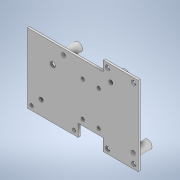
# Autodesk Inventor part: 10_Holder_Step_Down
Saved by Autodesk Inventor 2021 (Build 250183000, 183)
## iProperties
Created: 2021-07-29
Part Number: 10_Holder_Step_Down
Material: Generisch
Document SubType Name: Modeling
Designer: User
Density: 1 g/cm^3
Appearance: Vorgabe
Author: User
Autodesk Inventor part; units mm, degrees
ref_plane "YZ Plane" through (0, 0, 0) normal (1, 0, 0) x (0, 1, 0)
ref_plane "Arbeitsebene1" through (0, 0, 10) normal (0, 0, 1) x (1, 0, 0)
sketch "Skizze1" plane through (0, 0, 10) normal (0, 0, 1) x (1, 0, 0)
  circle A0 centre (19, -33.7337) radius 2 projected
  circle A1 centre (37, -73.7337) radius 2 projected
  circle A2 centre (-37, -73.7337) radius 2 projected
  circle A3 centre (-19, -33.7337) radius 2 projected
  circle A4 centre (37.3592, -81.4668) radius 1.25 projected
  circle A5 centre (16.3592, -81.4668) radius 1.25 projected
  circle A6 centre (16.3592, -24.9668) radius 1.25 projected
  circle A7 centre (37.3592, -24.9668) radius 1.25 projected
  circle A8 centre (9.1592, -42.7989) radius 0.8 projected
  circle A9 centre (-3.6408, -42.7989) radius 0.8 projected
  circle A10 centre (-3.6408, -70.7989) radius 0.8 projected
  circle A11 centre (9.1592, -70.7989) radius 0.8 projected
  circle A12 centre (-44.8022, -81.878) radius 1 projected
  circle A13 centre (-10.6794, -81.878) radius 1 projected
  circle A14 centre (-27.7408, -44.8166) radius 1.5 projected
  line L0 (40.9592, -85.0668) -> (40.9592, -21.3668)
  line L1 (40.9592, -21.3668) -> (12.7592, -21.3668)
  line L2 (12.7592, -21.3668) -> (12.7592, -29.3166)
  line L3 (12.7592, -29.3166) -> (-48.2408, -29.3166)
  line L4 (-48.2408, -29.3166) -> (-48.2408, -85.3166)
  line L5 (40.9592, -85.0668) -> (12.7592, -85.0668)
  line L6 (12.7592, -85.0668) -> (12.7592, -75.3989)
  line L7 (12.7592, -75.3989) -> (-7.2408, -75.3989)
  line L8 (-7.2408, -75.3989) -> (-7.2408, -85.3166)
  line L9 (-7.2408, -85.3166) -> (-48.2408, -85.3166)
  line L10 (39.9592, -84.0668) -> (39.9592, -22.3668) projected
  line L11 (39.9592, -22.3668) -> (13.7592, -22.3668) projected
  line L12 (13.7592, -84.0668) -> (39.9592, -84.0668) projected
  line L13 (13.7592, -22.3668) -> (13.7592, -84.0668) projected
  line L14 (-7.2408, -74.3989) -> (12.7592, -74.3989) projected
  line L15 (-47.2408, -84.3166) -> (-8.2408, -84.3166) projected
  line L16 (-47.2408, -37.3166) -> (-47.2408, -84.3166) projected
  line L17 (-31.0408, -31.3166) -> (-46.2408, -31.3166) projected
  line L18 (-8.2408, -84.3166) -> (-8.2408, -37.3166) projected
  circle A15 centre (-44.8022, -81.878) radius 1
  circle A16 centre (-27.7408, -44.8166) radius 1.7
  circle A17 centre (-3.6408, -42.7989) radius 1
  circle A18 centre (9.1592, -42.7989) radius 1
  circle A19 centre (-10.6794, -81.878) radius 1
  circle A20 centre (-3.6408, -70.7989) radius 1
  circle A21 centre (9.1592, -70.7989) radius 1
  circle A22 centre (16.3592, -81.4668) radius 1.45
  circle A23 centre (37.3592, -81.4668) radius 1.45
  circle A24 centre (37.3592, -24.9668) radius 1.45
  circle A25 centre (16.3592, -24.9668) radius 1.45
  circle A26 centre (19, -33.7337) radius 1.5753
  circle A27 centre (-19, -33.7337) radius 1.5753
  circle A28 centre (37, -73.7337) radius 1.5753
  circle A29 centre (-37, -73.7337) radius 1.5753
  point P0 (0, 0)
  dimension "d0" = 1
  dimension "d1" = 1
  dimension "d2" = 1
  dimension "d3" = 1
  dimension "d4" = 1
  dimension "d5" = 1
  dimension "d6" = 1
  dimension "d7" = 2
  dimension "d8" = 1
  dimension "d9" = 1
  dimension "d18" = 2
  dimension "d19" = 0.2
  dimension "d20" = 0.2
  dimension "d21" = 0.2
  dimension "d22" = 2
  dimension "d23" = 2
  dimension "d24" = 2
  dimension "d25" = 2
  dimension "d26" = 2
  dimension "d27" = 0.2
  dimension "d28" = 0.2
  dimension "d29" = 3.1505
  constraints: 20 end point, 15 centre point, 15 coincident, 8 perpendicular, 3 equal radius, 1 horizontal, 1 vertical
  measures "d0" distance between parallel lines of L0 L10
  measures "d1" distance between parallel lines of L5 L12
  measures "d2" distance between parallel lines of L13 L6
  measures "d3" distance between parallel lines of L14 L7
  measures "d4" distance between parallel lines of L8 L18
  measures "d5" distance between parallel lines of L9 L15
  measures "d6" distance between parallel lines of L16 L4
  measures "d7" distance between parallel lines of L17 L3
  measures "d8" distance between parallel lines of L13 L2
  measures "d9" distance between parallel lines of L11 L1
  measures "d18" diameter of A15
  measures "d19" radial gap between concentric circles of A14 A16
  measures "d20" radial gap between concentric circles of A6 A25
  measures "d21" radial gap between concentric circles of A7 A24
  measures "d22" diameter of A19
  measures "d23" diameter of A17
  measures "d24" diameter of A20
  measures "d25" diameter of A21
  measures "d26" diameter of A18
  measures "d27" radial gap between concentric circles of A5 A22
  measures "d28" radial gap between concentric circles of A4 A23
  measures "d29" diameter of A26
extrude "Extrusion1" add sketch "Skizze1" along normal blind 1.6 contours A0 | A1 | A2 | A3 | L5 L6 L7 L8 L9 L4 L3 L2 L1 L0 | L12 L13 L11 L10
sketch "Skizze2" plane through (0, 0, 10) normal (0, 0, -1) x (-1, 0, 0)
  circle A0 centre (-19, -33.7337) radius 3.4952
  circle A1 centre (19, -33.7337) radius 3.4952
  line L0 (-40.9592, -85.0668) -> (-40.9592, -21.3668) projected
  circle A2 centre (-19, -33.7337) radius 1.5752 projected
  circle A3 centre (19, -33.7337) radius 1.5752 projected
  circle A4 centre (-37, -73.7337) radius 3.4952
  circle A5 centre (-37, -73.7337) radius 1.5752 projected
  circle A6 centre (37, -73.7337) radius 1.5752 projected
  circle A7 centre (37, -73.7337) radius 3.4952
  circle A8 centre (-19, -33.7337) radius 1.5752 projected
  circle A9 centre (19, -33.7337) radius 1.5752 projected
  point P0 (0, 0)
  dimension "d30" = 1.92
  dimension "d31" = 1.92
  dimension "d32" = 1.92
  dimension "d33" = 1.92
  constraints: 8 coincident, 4 centre point
  measures "d30" radial gap between concentric circles of A0 A2
  measures "d31" radial gap between concentric circles of A3 A1
  measures "d32" radial gap between concentric circles of A4 A5
  measures "d33" radial gap between concentric circles of A7 A6
extrude "Extrusion2" add sketch "Skizze2" along normal blind 10
ref_plane "Arbeitsebene2" through (0, 0, -10) normal (0.8937807, 0.4485042, 0) x (0, 0, 1)
chamfer "Fase1" distance 0.5 angle 45 4 edges at (38.5753, -73.7337, 0) (20.5753, -33.7337, 0) (-17.4248, -33.7337, 0) (-35.4248, -73.7337, 0)
sketch "Skizze6" plane through (37, -73.7337, 0) normal (0, 0, -1) x (-1, 0, 0)
  circle A0 centre (0, 0) radius 3.4952 projected
  circle A1 centre (18, 40) radius 3.4952 projected
  circle A2 centre (56, 40) radius 3.4952 projected
  circle A3 centre (74, 0) radius 3.4952 projected
  circle A4 centre (56, 40) radius 1.5752 projected
  circle A5 centre (18, 40) radius 1.5752 projected
  point P0 (37, 73.7337)
  constraints: 4 coincident
sketch "Skizze5" plane through (0, 0, -10) normal (0.8937807, 0.4485042, 0) x (0, 0, 1)
  line L0 (9.55, 84.0717) -> (9.7375, 84.3964)
  line L1 (9.7375, 84.3964) -> (9.8125, 84.3964)
  line L2 (9.8125, 84.3964) -> (10, 84.0717)
  line L3 (10, 84.0717) -> (10.075, 84.0717)
  line L4 (10.15, 84.0717) -> (10.15, 84.4614) construction
  line L5 (10.15, 84.4614) -> (9.4, 84.4614) construction
  line L6 (9.4, 84.4614) -> (9.4, 84.0717) construction
  line L7 (9.4, 84.0717) -> (9.475, 84.0717) construction
  line L8 (9.475, 84.0717) -> (9.55, 84.0717)
  line L9 (10.075, 84.0717) -> (10.15, 84.0717) construction
  line L10 (9.55, 84.0717) -> (10, 84.0717) construction
  line L11 (9.7375, 84.3964) -> (9.775, 84.4614) construction
  line L12 (9.8125, 84.3964) -> (9.775, 84.4614) construction
  line L13 (9.4, 82.4964) -> (10.15, 82.4964) construction
  line L14 (9.4, 84.0717) -> (9.475, 83.9418) construction
  line L15 (9.475, 83.9418) -> (9.55, 84.0717) construction
  line L16 (10, 84.0717) -> (10.075, 83.9418) construction
  line L17 (10.075, 83.9418) -> (10.15, 84.0717) construction
  line L18 (9.775, 84.0717) -> (9.775, 84.4614) construction
  line L19 (9.475, 83.9418) -> (10.075, 83.9418) construction
  line L20 (9.4, 82.4964) -> (9.4, 84.0717) construction
  line L21 (10.15, 82.4964) -> (10.15, 84.0717) construction
  line L22 (9.55, 84.0717) -> (10, 84.0717)
  line L23 (25.04, 82.4964) -> (0.96, 82.4964) projected
  line L24 (10, 80.9212) -> (10, 84.0717) projected
  dimension "d34" = 60
  dimension "d35" = 3.8
  dimension "d36" = 0.6
  dimension "d37" = 3.1505
  dimension "d38" = 0.3247
  dimension "d39" = 0.0649
  constraints: 46 end point, 11 collinear, 5 parallel, 3 midpoint, 3 perpendicular, 3 point on line, 2 coincident, 1 horizontal, 9 other
  measures "d34" angle of L0 L2
  measures "d35" diameter of L0.end L13
  measures "d36" distance of L7.end L3.end
  measures "d37" diameter of L7.end L13
  measures "d38" distance between parallel lines of L1 L10
  measures "d39" distance from line of L18.end L1
coil "Spirale1" sketch "Skizze5" operation cut axis through (37, -73.7337, 10) along (0, 0, 1) pitch 0.6 turns 16.666667 hand right
pattern_sketch "Skizzenbasierte Anordnung1" of "Spirale1" from (37, -73.7337, 0) copies at (-19, -33.7337, 0) at (19, -33.7337, 0) at (-37, -73.7337, 0)
chamfer "Fase2" distance 0.4 angle 45 22 edges at (35.9092, -81.4668, 10) (35.9092, -81.4668, 11.6) (35.9092, -24.9668, 10) (35.9092, -24.9668, 11.6) (14.9092, -81.4668, 10) (14.9092, -81.4668, 11.6) (8.1592, -70.7989, 10) (8.1592, -70.7989, 11.6) (-4.6408, -70.7989, 10) (-4.6408, -70.7989, 11.6) (-11.6794, -81.878, 10) (-11.6794, -81.878, 11.6) (-4.6408, -42.7989, 10) (-4.6408, -42.7989, 11.6) (8.1592, -42.7989, 10) (8.1592, -42.7989, 11.6) (-45.8022, -81.878, 10) (-45.8022, -81.878, 11.6) (-29.4408, -44.8166, 10) (-29.4408, -44.8166, 11.6) (14.9092, -24.9668, 11.6) (14.9092, -24.9668, 10)
sketch "Skizze7" plane through (0, 0, 11.6) normal (0, 0, 1) x (1, 0, 0)
  circle A0 centre (37.3592, -24.9668) radius 1.45 projected
  circle A1 centre (16.3592, -24.9668) radius 1.45 projected
  circle A2 centre (9.1592, -42.7989) radius 1 projected
  circle A3 centre (-3.6408, -42.7989) radius 1 projected
  circle A4 centre (-27.7408, -44.8166) radius 1.7 projected
  circle A5 centre (-3.6408, -70.7989) radius 1 projected
  circle A6 centre (9.1592, -70.7989) radius 1 projected
  circle A7 centre (16.3592, -81.4668) radius 1.45 projected
  circle A8 centre (37.3592, -81.4668) radius 1.45 projected
  circle A9 centre (-10.6794, -81.878) radius 1 projected
  circle A10 centre (-44.8022, -81.878) radius 1 projected
  circle A11 centre (37.3592, -24.9668) radius 2.45
  circle A12 centre (37.3592, -81.4668) radius 2.45
  circle A13 centre (16.3592, -81.4668) radius 1.45 projected
  circle A14 centre (16.3592, -81.4668) radius 2.45
  circle A15 centre (9.1592, -70.7989) radius 1 projected
  circle A16 centre (9.1592, -70.7989) radius 2
  circle A17 centre (9.1592, -42.7989) radius 2
  circle A18 centre (-3.6408, -42.7989) radius 2
  circle A19 centre (-3.6408, -70.7989) radius 2
  circle A20 centre (-44.8022, -81.878) radius 2
  circle A21 centre (-10.6794, -81.878) radius 1 projected
  circle A22 centre (-10.6794, -81.878) radius 2
  circle A23 centre (-27.7408, -44.8166) radius 2.7
  circle A24 centre (16.3592, -24.9668) radius 1.45 projected
  circle A25 centre (16.3592, -24.9668) radius 2.45
  point P0 (0, 0)
  dimension "d56" = 1
  dimension "d57" = 1
  dimension "d58" = 1
  dimension "d59" = 1
  dimension "d60" = 1
  dimension "d61" = 1
  dimension "d62" = 1
  dimension "d63" = 1
  dimension "d64" = 1
  dimension "d65" = 1
  dimension "d66" = 1
  constraints: 11 centre point, 11 coincident
  measures "d56" radial gap between concentric circles of A11 A0
  measures "d57" radial gap between concentric circles of A8 A12
  measures "d58" radial gap between concentric circles of A7 A14
  measures "d59" radial gap between concentric circles of A6 A16
  measures "d60" radial gap between concentric circles of A2 A17
  measures "d61" radial gap between concentric circles of A1 A25
  measures "d62" radial gap between concentric circles of A3 A18
  measures "d63" radial gap between concentric circles of A4 A23
  measures "d64" radial gap between concentric circles of A10 A20
  measures "d65" radial gap between concentric circles of A9 A22
  measures "d66" radial gap between concentric circles of A5 A19
equation "\"d1\" = d0"
equation "\"d2\" = d0"
equation "\"d3\" = d0"
equation "\"d4\" = d0"
equation "\"d5\" = d0"
equation "\"d6\" = d0"
equation "\"d8\" = d0"
equation "\"d9\" = d0"
equation "\"d29\" = d43"
equation "\"d31\" = d30"
equation "\"d32\" = d30"
equation "\"d33\" = d30"
equation "\"d34\" = d40"
equation "\"d35\" = d41"
equation "\"d36\" = d42"
equation "\"d37\" = d43"
equation "\"d39\" = 0.125 * d44"
equation "\"d45\" = d42"
equation "\"d57\" = d56"
equation "\"d58\" = d56"
equation "\"d59\" = d56"
equation "\"d60\" = d56"
equation "\"d61\" = d56"
equation "\"d62\" = d56"
equation "\"d63\" = d56"
equation "\"d64\" = d56"
equation "\"d65\" = d56"
equation "\"d66\" = d56"
equation "\"d40\" = 60deg"
equation "\"d41\" = 3.8"
equation "\"d42\" = 0.6"
equation "\"d43\" = d41 - 1.0825 * d42"
equation "\"d44\" = 0.866 * d42"
